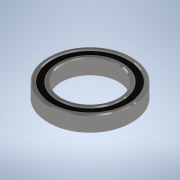
# Autodesk Inventor part: bearing 37x25x7
Saved by Autodesk Inventor 2022 (Build 260153000, 153)
## iProperties
Created: 2024-09-10
Part Number: bearing 37x25x7
Material: Типовые
Document SubType Name: Modeling
Designer: Andrey
Density: 1 g/cm^3
Appearance: Сталь — полированная
Author: Andrey
Autodesk Inventor part; units mm, degrees
ref_plane "YZ Plane" through (0, 0, 0) normal (1, 0, 0) x (0, 1, 0)
ref_plane "XZ Plane" through (0, 0, 0) normal (0, 1, 0) x (-1, 0, 0)
ref_plane "XY Plane" through (0, 0, 0) normal (0, 0, 1) x (1, 0, 0)
sketch "Эскиз1" plane through (0, 0, 0) normal (0, 1, 0) x (-1, 0, 0)
  circle A0 centre (0, 0) radius 12.5
  circle A1 centre (0, 0) radius 18.5
  dimension "d0" = 25
  dimension "d1" = 37
  constraints: 2 centre point, 2 coincident
  measures "d0" diameter of A0
  measures "d1" diameter of A1
extrude "Выдавливание1" add sketch "Эскиз1" along normal mid plane 7
sketch "Эскиз2" plane through (0, 3.5, 0) normal (0, 1, 0) x (1, 0, 0)
  circle A0 centre (0, 0) radius 14.2
  circle A1 centre (0, 0) radius 16.8
  circle A2 centre (0, 0) radius 12.5 projected
  dimension "d4" = 2.6
  dimension "d5" = 1.7
  constraints: 2 centre point, 1 coincident
  measures "d4" radial gap between concentric circles of A0 A1
  measures "d5" radial gap between concentric circles of A2 A0
extrude "Выдавливание2" cut sketch "Эскиз2" against normal blind 0.5 contours A1
chamfer "Фаска2" distance 0.4 angle 45 4 edges at (18.5, -3.5, 0) (18.5, 3.5, 0) (12.5, -3.5, 0) (12.5, 3.5, 0)
sketch "Эскиз3" plane through (0, -3.5, 0) normal (0, -1, 0) x (1, 0, 0)
  circle A0 centre (0, 0) radius 16.8 projected
  circle A1 centre (0, 0) radius 14.2 projected
extrude "Выдавливание3" cut sketch "Эскиз3" against normal blind 0.5
chamfer "Фаска1" distance 0.25 angle 45 4 edges at (-16.8, 3.5, 0) (-14.2, 3.5, 0) (-16.8, -3.5, 0) (-14.2, -3.5, 0)
